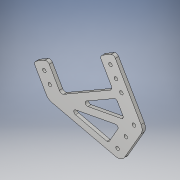
# Autodesk Inventor part: Part22
Saved by Autodesk Inventor 2019.4 (Build 234330000, 330)
## iProperties
Created: 2021-12-02
Part Number: Part22
Material: アルミニウム 6061
Document SubType Name: Modeling
Designer: 堀川皓史
Density: 2.7 g/cm^3
Appearance: アルミニウム - フラット
Author: 堀川皓史
Autodesk Inventor part; units mm, degrees
ref_plane "YZ Plane" through (0, 0, 0) normal (1, 0, 0) x (0, 1, 0)
ref_plane "XZ Plane" through (0, 0, 0) normal (0, 1, 0) x (-1, 0, 0)
ref_plane "XY Plane" through (0, 0, 0) normal (0, 0, 1) x (1, 0, 0)
sketch "スケッチ1" plane through (0, 0, 0) normal (0, 0, 1) x (1, 0, 0)
  line L0 (67.5, 17.5) -> (-67.5, 17.5) construction
  line L1 (-67.5, 17.5) -> (-67.5, -17.5) construction
  line L2 (-67.5, -17.5) -> (67.5, -17.5) construction
  line L3 (67.5, -17.5) -> (67.5, 17.5) construction
  line L4 (67.5, 17.5) -> (-67.5, -17.5) construction
  line L5 (-67.5, 17.5) -> (67.5, -17.5) construction
  circle A0 centre (-60, 35) radius 1.6 construction
  circle A1 centre (-70, 35) radius 1.6 construction
  line L6 (-77.5, 27.5) -> (-53, 27.5) construction
  line L7 (-53, 27.5) -> (-53, 42.5) construction
  line L8 (-53, 42.5) -> (-80, 42.5) construction
  line L9 (-77.5, 27.5) -> (-77.5, -27.5) construction
  line L10 (-77.5, -27.5) -> (-53, -27.5) construction
  line L11 (-53, -27.5) -> (-53, -42.5) construction
  line L12 (-53, -42.5) -> (-80, -42.5) construction
  circle A2 centre (-60, -35) radius 1.6 construction
  circle A3 centre (-70, -35) radius 1.6 construction
  circle A4 centre (-80, -35) radius 1.6 construction
  line L13 (124.2308, -31.7536) -> (484.5935, -392.1164)
  line L14 (484.5935, -392.1164) -> (488.7129, -553.575)
  line L15 (-80, 21.2868) -> (-468.838, -367.5512) construction
  line L16 (-468.838, -367.5512) -> (-479.4446, -356.9446)
  line L17 (-479.4446, -356.9446) -> (-90.6066, 31.8934) construction
  line L18 (-90.6066, 31.8934) -> (-80, 21.2868) construction
  line L19 (-80, 42.5) -> (-80, 5.3052) construction
  circle A5 centre (-92.3744, 19.519) radius 1.6 construction
  circle A6 centre (-102.981, 8.9124) radius 1.6 construction
  circle A7 centre (-113.5876, -1.6942) radius 1.6 construction
  line L20 (-92.3744, 19.519) -> (-113.5876, -1.6942) construction
  circle A8 centre (-437.941, -345.2067) radius 1.6
  circle A9 centre (-426.1402, -333.4059) radius 1.6
  line L21 (-388.4374, -772.2067) -> (-358.1265, -754.7067) construction
  line L22 (-358.1265, -754.7067) -> (-425.6265, -637.7933) construction
  line L23 (-455.9374, -655.2933) -> (-358.1265, -754.7067) construction
  line L24 (-388.4374, -772.2067) -> (-425.6265, -637.7933) construction
  line L25 (-455.9374, -655.2933) -> (-388.4374, -772.2067) construction
  line L26 (-425.6265, -637.7933) -> (-455.9374, -655.2933) construction
  line L27 (455.9374, -655.2933) -> (425.6265, -637.7933) construction
  line L28 (425.6265, -637.7933) -> (358.1265, -754.7067) construction
  line L29 (388.4374, -772.2067) -> (425.6265, -637.7933) construction
  line L30 (455.9374, -655.2933) -> (358.1265, -754.7067) construction
  line L31 (388.4374, -772.2067) -> (455.9374, -655.2933) construction
  line L32 (358.1265, -754.7067) -> (388.4374, -772.2067) construction
  line L33 (0, 0) -> (0, -263.4473) construction
  circle A10 centre (80, -35) radius 1.6 construction
  line L34 (67.5, 17.5) -> (67.5, -17.5) construction
  line L35 (77.5, 27.5) -> (53, 27.5) construction
  line L36 (77.5, 27.5) -> (77.5, -27.5) construction
  line L37 (77.5, -27.5) -> (53, -27.5) construction
  circle A11 centre (60, -35) radius 1.6 construction
  circle A12 centre (70, -35) radius 1.6 construction
  line L38 (53, -27.5) -> (53, -42.5) construction
  line L39 (53, -42.5) -> (80, -42.5) construction
  circle A13 centre (60, 35) radius 1.6 construction
  circle A14 centre (70, 35) radius 1.6 construction
  line L40 (80, 42.5) -> (80, 5.3052) construction
  line L41 (53, 42.5) -> (80, 42.5) construction
  line L42 (53, 27.5) -> (53, 42.5) construction
  line L43 (-392.0976, -785.867) -> (-404.3476, -764.6493)
  line L44 (-388.4374, -772.2067) -> (-358.1265, -754.7067) construction
  line L45 (-392.0976, -785.867) -> (-344.4662, -758.367)
  circle A15 centre (-336.7211, -756.782) radius 1.6
  circle A16 centre (-341.7211, -748.1218) radius 1.6
  line L46 (-343.7259, -729.6493) -> (-330.2259, -753.032)
  circle A17 centre (-346.7211, -739.4615) radius 1.6
  line L47 (-356.7162, -737.1493) -> (-343.7259, -729.6493)
  line L48 (-344.4662, -758.367) -> (-356.7162, -737.1493)
  circle A18 centre (-407.3428, -774.4615) radius 1.6
  circle A19 centre (-402.3428, -783.1218) radius 1.6
  line L49 (-404.3476, -764.6493) -> (-417.338, -772.1493)
  line L50 (-417.338, -772.1493) -> (-405.4634, -792.7168)
  line L51 (-403.838, -795.532) -> (-371.6264, -776.9346) construction
  line L52 (-425.6265, -637.7933) -> (-455.9374, -655.2933) construction
  line L53 (-409.7162, -645.3507) -> (-396.7259, -637.8507)
  circle A20 centre (-406.7211, -635.5385) radius 1.6
  line L54 (-455.9374, -655.2933) -> (-425.6265, -637.7933) construction
  circle A21 centre (-411.7211, -626.8782) radius 1.6
  line L55 (-469.5976, -651.633) -> (-421.9662, -624.133)
  line L56 (-421.9662, -624.133) -> (-409.7162, -645.3507)
  line L57 (-396.7259, -637.8507) -> (-410.2259, -614.468)
  circle A22 centre (-416.7211, -618.218) radius 1.6
  line L58 (-469.5976, -651.633) -> (-457.3476, -672.8507)
  circle A23 centre (-467.3428, -670.5385) radius 1.6
  circle A24 centre (-472.3428, -661.8782) radius 1.6
  line L59 (-483.838, -656.968) -> (-451.6264, -638.3706) construction
  line L60 (-470.338, -680.3507) -> (-483.838, -656.968)
  line L61 (-457.3476, -672.8507) -> (-470.338, -680.3507)
  line L62 (469.5976, -651.633) -> (457.3476, -672.8507)
  line L63 (455.9374, -655.2933) -> (425.6265, -637.7933) construction
  line L64 (469.5976, -651.633) -> (421.9662, -624.133)
  circle A25 centre (416.7211, -618.218) radius 1.6
  circle A26 centre (411.7211, -626.8782) radius 1.6
  line L65 (396.7259, -637.8507) -> (410.2259, -614.468)
  circle A27 centre (406.7211, -635.5385) radius 1.6
  line L66 (409.7162, -645.3507) -> (396.7259, -637.8507)
  line L67 (421.9662, -624.133) -> (409.7162, -645.3507)
  circle A28 centre (467.3428, -670.5385) radius 1.6
  circle A29 centre (472.3428, -661.8782) radius 1.6
  line L68 (457.3476, -672.8507) -> (470.338, -680.3507)
  line L69 (470.338, -680.3507) -> (483.838, -656.968)
  line L70 (483.838, -656.968) -> (451.6264, -638.3706) construction
  line L71 (358.1265, -754.7067) -> (388.4374, -772.2067) construction
  line L72 (356.7162, -737.1493) -> (343.7259, -729.6493)
  circle A30 centre (346.7211, -739.4615) radius 1.6
  line L73 (388.4374, -772.2067) -> (358.1265, -754.7067) construction
  circle A31 centre (341.7211, -748.1218) radius 1.6
  line L74 (392.0976, -785.867) -> (344.4662, -758.367)
  line L75 (344.4662, -758.367) -> (356.7162, -737.1493)
  line L76 (343.7259, -729.6493) -> (330.2259, -753.032)
  circle A32 centre (336.7211, -756.782) radius 1.6
  line L77 (392.0976, -785.867) -> (404.3476, -764.6493)
  circle A33 centre (407.3428, -774.4615) radius 1.6
  circle A34 centre (402.3428, -783.1218) radius 1.6
  line L78 (403.838, -795.532) -> (371.6264, -776.9346) construction
  line L79 (417.338, -772.1493) -> (403.838, -795.532)
  line L80 (404.3476, -764.6493) -> (417.338, -772.1493)
  line L81 (-483.838, -367.5512) -> (-468.838, -367.5512)
  line L82 (-468.838, -367.5512) -> (-468.838, -648.3077) construction
  line L83 (-468.838, -648.3077) -> (-483.838, -648.3077) construction
  line L84 (-483.838, -648.3077) -> (-483.838, -367.5512) construction
  line L85 (-283.2277, -604.4352) -> (-262.2277, -640.8083) construction
  line L86 (345.2492, -497.0108) -> (305.7786, -565.3759) construction
  line L87 (250, -655.004) -> (-250, -655.004) construction
  line L88 (-250, -655.004) -> (-250, -1155.004) construction
  line L89 (-250, -1155.004) -> (250, -1155.004) construction
  line L90 (250, -1155.004) -> (250, -655.004) construction
  line L91 (250, -655.004) -> (-250, -1155.004) construction
  line L92 (-250, -655.004) -> (250, -1155.004) construction
  line L93 (-12.841, -157.5) -> (15.1134, -157.5) construction
  circle A35 centre (-3.0548, -432.807) radius 212.5 construction
  line L94 (496.9452, 30.2659) -> (-503.0548, 30.2659) construction
  line L95 (-503.0548, 30.2659) -> (-503.0548, -969.7341) construction
  line L96 (-503.0548, -969.7341) -> (496.9452, -969.7341) construction
  line L97 (496.9452, -969.7341) -> (496.9452, 30.2659) construction
  line L98 (496.9452, 30.2659) -> (-503.0548, -969.7341) construction
  line L99 (-503.0548, 30.2659) -> (496.9452, -969.7341) construction
  circle A36 centre (-3.0548, -432.807) radius 250 construction
  line L100 (-80, 42.5) -> (-90.6066, 31.8934) construction
  line L101 (-80, 42.5) -> (-118.8909, 3.6091) construction
  line L102 (-118.8909, -6.2904) -> (-113.234, -11.9472) construction
  line L103 (-113.234, -11.9472) -> (-85.3433, -40.263) construction
  arc A37 (-118.8909, 3.6091) -> (-118.8909, -6.2904) centre (-113.9411, -1.3406) ccw construction
  arc A38 (-85.3433, -40.263) -> (-80, -42.5) centre (-80, -35) ccw construction
  line L104 (-80, 42.5) -> (-53, 42.5) construction
  circle A39 centre (-476.338, -638.3077) radius 1.6
  circle A40 centre (-476.338, -623.3077) radius 1.6
  circle A41 centre (-476.338, -608.2553) radius 1.6
  line L105 (-483.838, -656.968) -> (-483.838, -601.2553)
  line L106 (-483.838, -601.2553) -> (-468.838, -601.2553)
  line L107 (-468.838, -601.2553) -> (-415.3976, -610.8357)
  arc A42 (-410.2259, -614.468) -> (-415.3976, -610.8357) centre (-416.7211, -618.218) ccw
  line L108 (-255, -181.8915) -> (-270, -181.8915)
  line L109 (-270, -181.8915) -> (-270, -631.0383) construction
  line L110 (-270, -666.0383) -> (-255, -666.0383) construction
  line L111 (-255, -666.0383) -> (-255, -181.8915) construction
  line L112 (-271.0048, -667.7787) -> (-287.7211, -696.7321)
  line L113 (-426.5432, -937.1791) -> (-415.5605, -943.52)
  line L114 (-257.0096, -673.5383) -> (-270, -666.0383) construction
  line L115 (-325.2259, -761.6923) -> (-338.2162, -769.1923) construction
  circle A43 centre (-325.2259, -776.6923) radius 1.6
  circle A44 centre (-332.7259, -789.6827) radius 1.6
  circle A45 centre (-340.2259, -802.673) radius 1.6
  line L116 (-325.2259, -776.6923) -> (-340.2259, -802.673) construction
  line L117 (-330.2259, -753.032) -> (-318.7307, -772.9423)
  line L118 (-318.7307, -780.4423) -> (-333.7307, -806.423)
  line L119 (-400.6724, -796.2707) -> (-341.93, -809.9769)
  arc A46 (-405.4634, -792.7168) -> (-400.6724, -796.2707) centre (-398.9682, -788.9668) ccw
  arc A47 (-341.93, -809.9769) -> (-333.7307, -806.423) centre (-340.2259, -802.673) ccw
  arc A48 (-318.7307, -780.4423) -> (-318.7307, -772.9423) centre (-325.2259, -776.6923) ccw
  circle A49 centre (-268.7259, -678.8314) radius 1.6
  circle A50 centre (-276.2259, -691.8218) radius 1.6
  line L120 (-268.7259, -678.8314) -> (-283.7259, -704.8122) construction
  circle A51 centre (-262.5, -656.0383) radius 1.6
  circle A52 centre (-262.5, -641.0383) radius 1.6
  line L121 (-270, -631.0383) -> (-255, -631.0383)
  line L122 (-287.7211, -696.7321) -> (-274.7307, -704.2321)
  line L123 (-274.7307, -704.2321) -> (-257.0096, -673.5383)
  line L124 (-255, -631.0383) -> (-255, -666.0383)
  arc A53 (-257.0096, -673.5383) -> (-255, -666.0383) centre (-270, -666.0383) ccw
  line L125 (-270, -631.0383) -> (-270, -664.0287)
  line L126 (-287.7211, -696.7321) -> (-426.5432, -937.1791) construction
  arc A54 (-271.0048, -667.7787) -> (-270, -664.0287) centre (-277.5, -664.0287) ccw
  point P0 (-77.5, 0)
  point P1 (0, -470)
  point P2 (-123.8406, -1.3406)
  point P3 (-102.981, 8.9124)
  point P4 (-407.0319, -705)
  point P5 (-407.0319, -705)
  point P6 (407.0319, -705)
  point P7 (407.0319, -705)
  point P8 (77.5, 0)
  point P9 (-368.2819, -772.117)
  point P10 (-385.4668, -784.9254)
  point P11 (-445.7819, -637.883)
  point P12 (445.7819, -637.883)
  point P13 (465.4668, -646.3614)
  point P14 (368.2819, -772.117)
  point P15 (0, -905.004)
  point P16 (-3.0548, -469.7341)
  point P17 (0, -905.004)
  point P18 (-262.5, -666.0383)
  dimension "d4" = 135
  dimension "d5" = 35
  dimension "d6" = 3.2
  dimension "d7" = 3.2
  dimension "d8" = 10
  dimension "d9" = 15
  dimension "d10" = 10
  dimension "d11" = 7.5
  dimension "d12" = 7
  dimension "d13" = 70
  dimension "d14" = 3.2
  dimension "d15" = 3.2
  dimension "d16" = 3.2
  dimension "d17" = 10
  dimension "d18" = 10
  dimension "d19" = 7
  dimension "d20" = 15
  dimension "d21" = 7.5
  dimension "d22" = 10
  dimension "d23" = 10
  dimension "d24" = 135
  dimension "d25" = 15
  dimension "d26" = 10
  dimension "d27" = 3.2
  dimension "d28" = 3.2
  dimension "d29" = 3.2
  dimension "d30" = 10
  dimension "d31" = 15
  dimension "d32" = 15
  dimension "d33" = 7.5
  dimension "d34" = 45
  dimension "d35" = 3.2
  dimension "d36" = 3.2
  dimension "d37" = 360
  dimension "d38" = 360
  dimension "d39" = 470
  dimension "d40" = 15
  dimension "d41" = 200
  dimension "d42" = 200
  dimension "d43" = 500
  dimension "d44" = 500
  dimension "d45" = 200
  dimension "d46" = 425
  dimension "d47" = 1000
  dimension "d48" = 1000
  dimension "d49" = 42
  dimension "d50" = 500
  dimension "d51" = 7
  dimension "d52" = 7
  dimension "d53" = 3.2
  dimension "d54" = 3.2
  dimension "d55" = 3.2
  dimension "d56" = 15
  dimension "d57" = 15.0524
  dimension "d58" = 7.5
  dimension "d59" = 10
  dimension "d60" = 7
  dimension "d61" = 15
  dimension "d62" = 5
  dimension "d64" = 150
  dimension "d65" = 10
  dimension "d66" = 15
  dimension "d67" = 3.2
  dimension "d68" = 3.2
  constraints: 254 end point, 55 centre point, 23 parallel, 19 midpoint, 19 perpendicular, 18 point on line, 16 point on circle, 16 symmetric about line, 14 tangent, 9 coincident, 9 horizontal, 8 vertical alignment, 3 collinear, 3 horizontal alignment, 3 vertical, 2 equal radius, 242 other
  measures "d4" distance of L2.end L1.end
  measures "d5" distance of L1.end L0.end
  measures "d6" diameter of A0
  measures "d7" diameter of A1
  measures "d8" distance of A0.centre A1.centre
  measures "d9" distance between parallel lines of L6 L8
  measures "d10" distance between parallel lines of L0 L6
  measures "d11" distance from line of L6 A0.centre
  measures "d12" distance from line of L7 A0.centre
  measures "d13" horizontal distance of A1.centre point (0, 0)
  measures "d14" diameter of A2
  measures "d15" diameter of A3
  measures "d16" diameter of A4
  measures "d17" distance of A3.centre A4.centre
  measures "d18" distance of A2.centre A3.centre
  measures "d19" distance from line of L11 A2.centre
  measures "d20" distance between parallel lines of L12 L10
  measures "d21" distance from line of L12 A2.centre
  measures "d22" distance between parallel lines of L10 L2
  measures "d23" distance between parallel lines of L9 L1
  measures "d24" angle of L2 L13
  measures "d25" distance of L15.end L16.end
  measures "d26" distance from line of A1.centre L19
  measures "d27" diameter of A5
  measures "d28" diameter of A6
  measures "d29" diameter of A7
  measures "d30" distance from line of L18 L20.start
  measures "d31" distance of A6.centre L20.start
  measures "d32" distance of L20.end A6.centre
  measures "d33" distance between parallel lines of L15 L20
  measures "d34" angle of L9 L15
  measures "d35" diameter of A8
  measures "d36" diameter of A9
  measures "d39" distance of point (0, -470) point (-407.032, -705)
  measures "d40" distance of L82.end L83.end
  measures "d41" distance between parallel lines of L50 L85
  measures "d42" distance between parallel lines of L79 L86
  measures "d43" distance of L89.end L88.end
  measures "d44" distance of L88.end L87.end
  measures "d45" distance from line of L93.end L8
  measures "d46" diameter of A35
  measures "d47" distance of L96.end L95.end
  measures "d48" distance of L95.end L94.end
  measures "d49" distance of L85.start L85.end
  measures "d50" diameter of A36
  measures "d51" distance from line of L102 L20.end
  measures "d52" radius of A37
  measures "d53" diameter of A39
  measures "d54" diameter of A40
  measures "d55" diameter of A41
  measures "d56" distance of A40.centre A39.centre
  measures "d57" distance of A41.centre A40.centre
  measures "d58" distance from line of L84 A39.centre
  measures "d59" distance from line of L83 A39.centre
  measures "d60" distance from line of A41.centre L106
  measures "d61" distance of L110.start L110.end
  measures "d62" distance between parallel lines of L88 L111
  measures "d64" angle of L112 L109
  measures "d65" distance from line of L115 A15.centre
  measures "d66" distance of L115.start L115.end
  measures "d67" diameter of A43
  measures "d68" diameter of A44
extrude "押し出し1" add sketch "スケッチ1" along normal blind 3 contours L45 L48 L47 L46 L117 A48 L118 A47 L119 A46 L50 L49 L43
fillet "フィレット1" radius 3 6 edges at (-417.338, -772.1493, 1.5) (-404.3476, -764.6493, 1.5) (-392.0976, -785.867, 1.5) (-344.4662, -758.367, 1.5) (-356.7162, -737.1493, 1.5) (-343.7259, -729.6493, 1.5)
sketch "スケッチ2" plane through (0, 0, 3) normal (0, 0, 1) x (1, 0, 0)
  line L0 (-388.0069, -793.0647) -> (-348.6417, -802.2497)
  line L1 (-348.6417, -802.2497) -> (-337.8456, -783.5503)
  line L2 (-337.8456, -783.5503) -> (-388.0069, -793.0647)
  line L3 (-379.0415, -785.2572) -> (-333.8861, -776.6923)
  line L4 (-333.8861, -776.6923) -> (-341.4662, -763.5631)
  line L5 (-341.4662, -763.5631) -> (-379.0415, -785.2572)
  line L6 (-347.0643, -759.867) -> (-389.4996, -784.367) projected
  line L7 (-400.6724, -796.2707) -> (-341.93, -809.9769) projected
  line L8 (-333.7307, -806.423) -> (-318.7307, -780.4423) projected
  line L9 (-318.7307, -772.9423) -> (-342.2259, -732.2474) projected
  circle A0 centre (-407.3428, -774.4615) radius 1.6 construction
  line L10 (-407.3428, -774.4615) -> (-397.3428, -791.782) construction
  circle A1 centre (-402.3428, -783.1218) radius 1.6 construction
  line L11 (-378.9734, -788.2978) -> (-397.3428, -791.782) construction
  point P0 (0, 0)
  dimension "d83" = 6
  dimension "d84" = 6
  dimension "d86" = 15
  dimension "d87" = 15
  dimension "d88" = 6
  dimension "d89" = 10
  dimension "d90" = 3
  constraints: 16 end point, 6 parallel, 1 midpoint, 1 point on line
  measures "d83" distance between parallel lines of L7 L0
  measures "d84" distance between parallel lines of L6 L5
  measures "d86" distance between parallel lines of L8 L1
  measures "d87" distance between parallel lines of L9 L4
  measures "d88" distance between parallel lines of L2 L3
  measures "d89" distance of A1.centre L10.end
  measures "d90" distance between parallel lines of L3 L11
extrude "押し出し2" cut sketch "スケッチ2" against normal blind 3
fillet "フィレット2" radius 2 6 edges at (-341.4662, -763.5631, 1.5) (-333.8861, -776.6923, 1.5) (-379.0415, -785.2572, 1.5) (-388.0069, -793.0647, 1.5) (-348.6417, -802.2497, 1.5) (-337.8456, -783.5503, 1.5)
